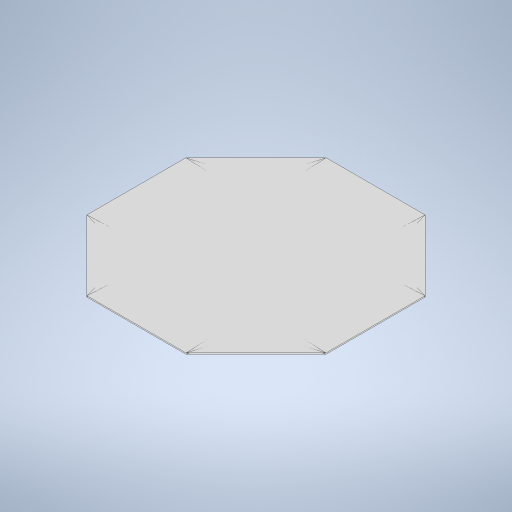
# Autodesk Inventor part: 팔각형 OV-PAM 층 한개
Saved by Autodesk Inventor 2024 (Build 280153000, 153)
## iProperties
Created: 2023-06-16
Part Number: 팔각형 OV-PAM 층 한개
Material: 일반
Document SubType Name: Modeling
Designer: jsw
Density: 1 g/cm^3
Appearance: 기본값
Mass: 0.852596 g
Surface Area: 109.11 cm^2
Volume: 0.852596 cm^3
Author: jsw
Autodesk Inventor part; units mm, degrees
sketch "스케치1" plane through (0, 0, 0) normal (0, 1, 0) x (-1, 0, 0)
  line L0 (-31.7919, 13.1686) -> (-13.1686, 31.7919)
  line L1 (-13.1686, 31.7919) -> (13.1686, 31.7919)
  line L2 (13.1686, 31.7919) -> (31.7919, 13.1686)
  line L3 (31.7919, 13.1686) -> (31.7919, -13.1686)
  line L4 (31.7919, -13.1686) -> (13.1686, -31.7919)
  line L5 (13.1686, -31.7919) -> (-13.1686, -31.7919)
  line L6 (-13.1686, -31.7919) -> (-31.7919, -13.1686)
  line L7 (-31.7919, -13.1686) -> (-31.7919, 13.1686)
  line L8 (-13.5, 32.5919) -> (13.5, 32.5919)
  line L9 (13.5, 32.5919) -> (32.5919, 13.5)
  line L10 (32.5919, 13.5) -> (32.5919, -13.5)
  line L11 (32.5919, -13.5) -> (13.5, -32.5919)
  line L12 (13.5, -32.5919) -> (-13.5, -32.5919)
  line L13 (-13.5, -32.5919) -> (-32.5919, -13.5)
  line L14 (-32.5919, -13.5) -> (-32.5919, 13.5)
  line L15 (-32.5919, 13.5) -> (-13.5, 32.5919)
  point P0 (0, 0)
  point P1 (0, 0)
  point P2 (0, 0)
  dimension "d2" = 0.8
  dimension "d42" = 27
  constraints: 32 end point, 2 coincident, 2 horizontal, 34 other
  measures "d2" distance between parallel lines of L10 L3
  measures "d42" distance of L11.end L12.end
extrude "돌출2" add sketch "스케치1" along normal blind 0.1612 contours L0 L1 L2 L3 L4 L5 L6 L7 | L8 L9 L10 L11 L12 L13 L14 L15
ref_plane "작업 평면2" through (32.5919, 0, 13.5) normal (-0.0174524, -0.9998477, 0) x (0, 0, -1)
sketch "스케치3" plane through (32.5919, 0, 13.5) normal (1, 0, 0) x (0, 0, -1)
  line L0 (0, 0) -> (0, 0.1612) projected
  line L1 (0, 0.1612) -> (27, 0.1612) projected
  line L2 (0, 0) -> (27, 0)
  line L3 (27, 0) -> (27, 0.1612)
  line L4 (27, 0.1612) -> (0, 0.1612)
  line L5 (0, 0.1612) -> (0, 0)
  line L6 (0, 0.1612) -> (-92.371, 0.1612)
  line L7 (-19.0919, 0.1612) -> (0, 0.1612) projected
  line L8 (0, 0) -> (-92.371, 0.1612)
  line L9 (27, 0.1612) -> (119.371, 0.1612)
  line L10 (119.371, 0.1612) -> (27, 0)
  point P0 (13.5, 0)
  dimension "d17" = 179.9
  dimension "d18" = 179.9
  constraints: 16 end point, 2 parallel, 2 point on line, 1 horizontal, 1 perpendicular
  measures "d17" angle of L8 L2
  measures "d18" angle of L2 L10
extrude "돌출4" cut sketch "스케치3" against normal up to surface surface through (32.5919, 0, 13.5) normal (-0.0174524, -0.9998477, 0)
sketch "스케치4" plane through (13.5, 0, 32.5919) normal (0.7071068, 0, 0.7071068) x (0.7071068, 0, -0.7071068)
  line L0 (0, 0) -> (0, 0.1612) projected
  line L1 (27, 0) -> (27, 0.1612) projected
  line L2 (0, 0) -> (27, 0)
  line L3 (27, 0) -> (27, 0.1612)
  line L4 (27, 0.1612) -> (0, 0.1612)
  line L5 (0, 0.1612) -> (0, 0)
  line L6 (27, 0) -> (13.9381, 0.1612) projected
  line L7 (27, 0) -> (18.609, 0.1612)
  line L8 (27, 0) -> (0, 0) projected
  line L9 (0, 0) -> (8.391, 0.1612)
  line L10 (27, 0.1612) -> (0, 0.1612) projected
  point P0 (13.5, 0)
  point P1 (8.391, 0.1612)
  point P2 (13.5, 0.1612)
  dimension "d40" = 10.218
  dimension "d41" = 5.109
  constraints: 12 end point, 2 parallel, 2 point on line, 1 horizontal, 1 midpoint, 1 perpendicular, 1 other
  measures "d40" distance of L9.end L7.end
  measures "d41" distance of point (13.5, 0.161) L7.end
ref_plane "작업 평면3" through (13.5, 0, 32.5919) normal (0.0123407, 0.9998477, 0.0123407) x (0.7071068, 0, -0.7071068)
extrude "돌출5" cut sketch "스케치4" against normal up to surface contours L9 L4 L6 L2 | L6 L4 L7 surface through (13.5, 0, 32.5919) normal (0.0123407, 0.9998477, 0.0123407)
pattern_circular "원형 패턴1" count 4 over 360 about axis through (0, -10, 0) along (0, 1, 0) of "돌출4"
pattern_circular "원형 패턴2" count 4 over 360 about axis through (0, -10, 0) along (0, 1, 0) of "돌출5"
mirror "미러5" about plane through (0, 0.1612, 0) normal (0, 1, 0) of "돌출2", "돌출5", "원형 패턴2", "돌출4", "원형 패턴1"
ref_plane "작업 평면5" through (-13.5, 0.1612, -32.5919) normal (0, 1, 0) x (1, 0, 0)
equation "\"d41\" = 0.5 * d40"
